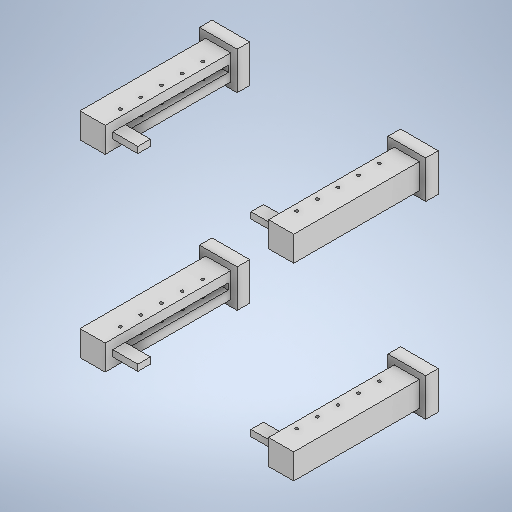
# Autodesk Inventor part: Torres
Saved by Autodesk Inventor 2026 (Build 300175050, 175E)
## iProperties
Created: 2025-04-14
Part Number: Torres
Material: Genérico
Document SubType Name: Modeling
Designer: piero
Density: 1 g/cm^3
Appearance: Valor por defecto
Author: piero
Autodesk Inventor part; units mm, degrees
ref_plane "YZ Plane" through (0, 0, 0) normal (1, 0, 0) x (0, 1, 0)
ref_plane "XZ Plane" through (0, 0, 0) normal (0, 1, 0) x (-1, 0, 0)
ref_plane "XY Plane" through (0, 0, 0) normal (0, 0, 1) x (1, 0, 0)
sketch "Boceto1" plane through (0, 0, 0) normal (0, 0, 1) x (1, 0, 0)
  line L0 (-82.5537, 351.7864) -> (67.4463, 351.7864)
  line L1 (67.4463, 351.7864) -> (67.4463, 201.7864)
  line L2 (67.4463, 201.7864) -> (-82.5537, 201.7864)
  line L3 (-82.5537, 201.7864) -> (-82.5537, 351.7864)
  line L4 (-82.5537, 351.7864) -> (67.4463, 201.7864) construction
  line L5 (67.4463, 351.7864) -> (-82.5537, 201.7864) construction
  line L6 (667.4463, 201.7864) -> (817.4463, 201.7864)
  line L7 (817.4463, 201.7864) -> (817.4463, 351.7864)
  line L8 (817.4463, 351.7864) -> (667.4463, 351.7864)
  line L9 (667.4463, 351.7864) -> (667.4463, 201.7864)
  line L10 (667.4463, 201.7864) -> (817.4463, 351.7864) construction
  line L11 (817.4463, 201.7864) -> (667.4463, 351.7864) construction
  line L12 (-82.5537, -548.2136) -> (67.4463, -548.2136)
  line L13 (67.4463, -548.2136) -> (67.4463, -398.2136)
  line L14 (67.4463, -398.2136) -> (-82.5537, -398.2136)
  line L15 (-82.5537, -398.2136) -> (-82.5537, -548.2136)
  line L16 (-82.5537, -548.2136) -> (67.4463, -398.2136) construction
  line L17 (67.4463, -548.2136) -> (-82.5537, -398.2136) construction
  line L18 (667.4463, -548.2136) -> (817.4463, -548.2136)
  line L19 (817.4463, -548.2136) -> (817.4463, -398.2136)
  line L20 (817.4463, -398.2136) -> (667.4463, -398.2136)
  line L21 (667.4463, -398.2136) -> (667.4463, -548.2136)
  line L22 (667.4463, -548.2136) -> (817.4463, -398.2136) construction
  line L23 (817.4463, -548.2136) -> (667.4463, -398.2136) construction
  point P0 (0, 0)
  point P1 (-7.5537, 276.7864)
  point P2 (742.4463, 276.7864)
  point P3 (-7.5537, -473.2136)
  point P4 (742.4463, -473.2136)
  point P5 (-7.5537, -398.2136)
  point P6 (742.4463, -398.2136)
  point P7 (667.4463, 276.7864)
  point P8 (667.4463, -473.2136)
  point P9 (67.4463, -473.2136)
  dimension "d0" = 150
  dimension "d1" = 150
  dimension "d2" = 150
  dimension "d3" = 150
  dimension "d4" = 150
  dimension "d5" = 150
  dimension "d6" = 150
  dimension "d7" = 150
  dimension "d8" = 600
  dimension "d9" = 600
  dimension "d10" = 600
  dimension "d11" = 600
  constraints: 48 end point, 13 midpoint, 8 parallel, 4 horizontal, 4 perpendicular
  measures "d0" distance of L1.end L2.end
  measures "d1" distance of L0.end L1.end
  measures "d2" distance of L8.end L7.end
  measures "d3" distance of L7.end L6.end
  measures "d4" distance of L14.end L13.end
  measures "d5" distance of L13.end L12.end
  measures "d6" distance of L20.end L19.end
  measures "d7" distance of L19.end L18.end
  measures "d8" distance from line of point (-7.554, -398.214) L2
  measures "d9" distance from line of point (742.446, -398.214) L6
  measures "d10" distance from line of point (667.446, 276.786) L1
  measures "d11" distance of point (667.446, -473.214) point (67.446, -473.214)
extrude "Extrusión1" add sketch "Boceto1" along normal blind 50
sketch "Boceto2" plane through (0, 0, 50) normal (0, 0, 1) x (1, 0, 0)
  line L0 (-57.5537, 326.7864) -> (42.4463, 326.7864)
  line L1 (42.4463, 326.7864) -> (42.4463, 226.7864)
  line L2 (42.4463, 226.7864) -> (-57.5537, 226.7864)
  line L3 (-57.5537, 226.7864) -> (-57.5537, 326.7864)
  line L4 (-57.5537, 326.7864) -> (42.4463, 226.7864) construction
  line L5 (42.4463, 326.7864) -> (-57.5537, 226.7864) construction
  line L6 (692.4463, 326.7864) -> (792.4463, 326.7864)
  line L7 (792.4463, 326.7864) -> (792.4463, 226.7864)
  line L8 (792.4463, 226.7864) -> (692.4463, 226.7864)
  line L9 (692.4463, 226.7864) -> (692.4463, 326.7864)
  line L10 (692.4463, 326.7864) -> (792.4463, 226.7864) construction
  line L11 (792.4463, 326.7864) -> (692.4463, 226.7864) construction
  line L12 (692.4463, -423.2136) -> (792.4463, -423.2136)
  line L13 (792.4463, -423.2136) -> (792.4463, -523.2136)
  line L14 (792.4463, -523.2136) -> (692.4463, -523.2136)
  line L15 (692.4463, -523.2136) -> (692.4463, -423.2136)
  line L16 (692.4463, -423.2136) -> (792.4463, -523.2136) construction
  line L17 (792.4463, -423.2136) -> (692.4463, -523.2136) construction
  line L18 (-57.5537, -523.2136) -> (42.4463, -523.2136)
  line L19 (42.4463, -523.2136) -> (42.4463, -423.2136)
  line L20 (42.4463, -423.2136) -> (-57.5537, -423.2136)
  line L21 (-57.5537, -423.2136) -> (-57.5537, -523.2136)
  line L22 (-57.5537, -523.2136) -> (42.4463, -423.2136) construction
  line L23 (42.4463, -523.2136) -> (-57.5537, -423.2136) construction
  line L24 (67.4463, 351.7864) -> (-82.5537, 351.7864) projected
  line L25 (-82.5537, 351.7864) -> (-82.5537, 201.7864) projected
  line L26 (817.4463, 351.7864) -> (667.4463, 351.7864) projected
  line L27 (667.4463, 351.7864) -> (667.4463, 201.7864) projected
  line L28 (817.4463, -398.2136) -> (667.4463, -398.2136) projected
  line L29 (-82.5537, -398.2136) -> (-82.5537, -548.2136) projected
  line L30 (67.4463, -398.2136) -> (-82.5537, -398.2136) projected
  point P0 (0, 0)
  point P1 (-7.5537, 276.7864)
  point P2 (742.4463, 276.7864)
  point P3 (742.4463, -473.2136)
  point P4 (-7.5537, -473.2136)
  point P5 (742.4463, 351.7864)
  point P6 (742.4463, 326.7864)
  point P7 (692.4463, 276.7864)
  dimension "d14" = 100
  dimension "d15" = 100
  dimension "d16" = 100
  dimension "d17" = 100
  dimension "d18" = 100
  dimension "d19" = 100
  dimension "d20" = 25
  dimension "d21" = 25
  dimension "d22" = 25
  dimension "d23" = 25
  dimension "d24" = 25
  dimension "d25" = 25
  dimension "d26" = 25
  constraints: 48 end point, 11 midpoint, 8 parallel, 4 horizontal, 4 perpendicular, 3 point on line
  measures "d14" distance of L1.end L2.end
  measures "d15" distance of L0.end L1.end
  measures "d16" distance of L7.end L8.end
  measures "d17" distance of L6.end L7.end
  measures "d18" distance of L13.end L14.end
  measures "d19" distance of L12.end L13.end
  measures "d20" distance between parallel lines of L24 L0
  measures "d21" distance between parallel lines of L25 L3
  measures "d22" distance of point (742.446, 351.786) point (742.446, 326.786)
  measures "d23" distance from line of L27 point (692.446, 276.786)
  measures "d24" distance between parallel lines of L28 L12
  measures "d25" distance between parallel lines of L29 L21
  measures "d26" distance between parallel lines of L20 L30
extrude "Extrusión2" add sketch "Boceto2" along normal blind 500
sketch "Boceto5" plane through (692.4463, 226.7864, 50) normal (-1, 0, 0) x (0, 0, 1)
  line L0 (470, 62.5) -> (420, 62.5) projected
  line L1 (470, 37.5) -> (470, 62.5) projected
  line L2 (420, 37.5) -> (470, 37.5) projected
  line L3 (420, 62.5) -> (420, 37.5) projected
  line L4 (420, 62.5) -> (470, 62.5) projected
  line L5 (470, 62.5) -> (10, 62.5)
  line L6 (10, 62.5) -> (10, 37.5)
  line L7 (10, 37.5) -> (470, 37.5)
  line L8 (470, 37.5) -> (470, 62.5)
  line L9 (470, -712.5) -> (470, -687.5) projected
  line L10 (470, -687.5) -> (10, -687.5)
  line L11 (10, -687.5) -> (10, -712.5)
  line L12 (10, -712.5) -> (470, -712.5)
  line L13 (470, -712.5) -> (470, -687.5)
  point P0 (-50, -226.7864)
  dimension "d41" = 460
  dimension "d42" = 460
  constraints: 16 end point, 4 parallel, 2 horizontal, 2 perpendicular, 1 point on line
  measures "d41" distance of L7.end L6.end
  measures "d42" distance of L12.end L11.end
extrude "Extrusión5" cut sketch "Boceto5" against normal blind 50
sketch "Boceto6" plane through (742.4463, 226.7864, 50) normal (-1, 0, 0) x (0, 0, 1)
  line L0 (470, 62.5) -> (470, 37.5) projected
  line L1 (470, 37.5) -> (10, 37.5) projected
  line L2 (470, 62.5) -> (420, 62.5)
  line L3 (420, 62.5) -> (420, 37.5)
  line L4 (420, 37.5) -> (470, 37.5)
  line L5 (470, 37.5) -> (470, 62.5)
  line L6 (10, -687.5) -> (470, -687.5) projected
  line L7 (470, -712.5) -> (10, -712.5) projected
  line L8 (470, -687.5) -> (420, -687.5)
  line L9 (420, -687.5) -> (420, -712.5)
  line L10 (420, -712.5) -> (470, -712.5)
  line L11 (470, -712.5) -> (470, -687.5)
  point P0 (-50, -226.7864)
  dimension "d45" = 50
  dimension "d46" = 50
  constraints: 16 end point, 4 parallel, 2 horizontal, 2 perpendicular, 2 point on line
  measures "d45" distance of L4.end L3.end
  measures "d46" distance of L10.end L9.end
extrude "Extrusión6" add sketch "Boceto6" along normal blind 150
sketch "Boceto7" plane through (42.4463, -523.2136, 50) normal (1, 0, 0) x (0, 0, -1)
  line L0 (-470, 37.5) -> (-420, 37.5) projected
  line L1 (-10, 62.5) -> (-420, 62.5) projected
  line L2 (-470, 37.5) -> (-10, 37.5)
  line L3 (-10, 37.5) -> (-10, 62.5)
  line L4 (-10, 62.5) -> (-470, 62.5)
  line L5 (-470, 62.5) -> (-470, 37.5)
  line L6 (-470, 787.5) -> (-420, 787.5) projected
  line L7 (-470, 787.5) -> (-10, 787.5)
  line L8 (-10, 787.5) -> (-10, 812.5)
  line L9 (-10, 812.5) -> (-470, 812.5)
  line L10 (-470, 812.5) -> (-470, 787.5)
  point P0 (50, 523.2136)
  dimension "d49" = 460
  dimension "d50" = 460
  constraints: 16 end point, 4 parallel, 2 horizontal, 2 perpendicular
  measures "d49" distance of L4.end L1.start
  measures "d50" distance of L9.end L8.end
extrude "Extrusión7" cut sketch "Boceto7" against normal blind 50
sketch "Boceto8" plane through (-7.5537, -523.2136, 50) normal (1, 0, 0) x (0, 0, -1)
  line L0 (-470, 62.5) -> (-470, 37.5) projected
  line L1 (-420, 62.5) -> (-470, 62.5) projected
  line L2 (-470, 37.5) -> (-420, 37.5)
  line L3 (-420, 37.5) -> (-420, 62.5)
  line L4 (-420, 62.5) -> (-470, 62.5)
  line L5 (-470, 62.5) -> (-470, 37.5)
  line L6 (-470, 787.5) -> (-420, 787.5) projected
  line L7 (-470, 812.5) -> (-420, 812.5) projected
  line L8 (-470, 787.5) -> (-420, 787.5)
  line L9 (-420, 787.5) -> (-420, 812.5)
  line L10 (-420, 812.5) -> (-470, 812.5)
  line L11 (-470, 812.5) -> (-470, 787.5)
  point P0 (50, 523.2136)
  dimension "d53" = 50
  dimension "d54" = 50
  constraints: 16 end point, 4 parallel, 2 horizontal, 2 perpendicular
  measures "d53" distance of L4.end L1.start
  measures "d54" distance of L10.end L7.end
extrude "Extrusión8" add sketch "Boceto8" along normal blind 150
sketch "Boceto9" plane through (-57.5537, -523.2136, 50) normal (0, -1, 0) x (1, 0, 0)
  line L0 (50, 420) -> (100, 420) projected
  circle A0 centre (74, 414) radius 6
  circle A1 centre (74, 332) radius 6
  circle A2 centre (74, 250) radius 6
  circle A3 centre (74, 168) radius 6
  circle A4 centre (74, 86) radius 6
  line L1 (100, 0) -> (100, 500) projected
  circle A5 centre (776, 414) radius 6
  line L2 (750, 420) -> (800, 420) projected
  line L3 (750, 0) -> (750, 500) projected
  circle A6 centre (776, 332) radius 6
  circle A7 centre (776, 250) radius 6
  circle A8 centre (776, 168) radius 6
  circle A9 centre (776, 86) radius 6
  line L4 (725, 0) -> (875, 0) projected
  point P0 (57.5537, -50)
  dimension "d60" = 12
  dimension "d61" = 0
  dimension "d62" = 12
  dimension "d63" = 70
  dimension "d64" = 12
  dimension "d65" = 12
  dimension "d66" = 12
  dimension "d69" = 82
  dimension "d70" = 70
  dimension "d71" = 82
  dimension "d74" = 20
  dimension "d75" = 12
  dimension "d76" = 0
  dimension "d77" = 20
  dimension "d78" = 12
  dimension "d83" = 82
  dimension "d84" = 12
  dimension "d85" = 82
  dimension "d86" = 12
  dimension "d87" = 70
  dimension "d88" = 12
  dimension "d89" = 82
  constraints: 10 centre point
  measures "d60" diameter of A0
  measures "d61" distance edge to line of A0 L0
  measures "d62" diameter of A1
  measures "d64" diameter of A2
  measures "d65" diameter of A3
  measures "d66" diameter of A4
  measures "d69" distance of A2.centre A1.centre
  measures "d71" distance of A4.centre A3.centre
  measures "d74" distance edge to line of A0 L1
  measures "d75" diameter of A5
  measures "d76" distance edge to line of A5 L2
  measures "d77" distance edge to line of A5 L3
  measures "d78" diameter of A6
  measures "d83" distance of A6.centre A5.centre
  measures "d84" diameter of A7
  measures "d85" distance of A7.centre A6.centre
  measures "d86" diameter of A8
  measures "d88" diameter of A9
  measures "d89" distance of A9.centre A8.centre
hole "Agujero1" at (16.4463, -523.2136, 464) direction (0, 1, 0) diameter 11.835 depth 100 thread size "M14x2" class "6H" standard "ISO Metric profile"
hole "Agujero2" at (16.4463, -523.2136, 382) direction (0, 1, 0) diameter 11.835 depth 100 thread size "M14x2" class "6H" standard "ISO Metric profile"
hole "Agujero3" at (16.4463, -523.2136, 300) direction (0, 1, 0) diameter 11.835 depth 100 thread size "M14x2" class "6H" standard "ISO Metric profile"
hole "Agujero4" at (16.4463, -523.2136, 218) direction (0, 1, 0) diameter 11.835 depth 100 thread size "M14x2" class "6H" standard "ISO Metric profile"
hole "Agujero5" at (16.4463, -523.2136, 136) direction (0, 1, 0) diameter 11.835 depth 100 thread size "M14x2" class "6H" standard "ISO Metric profile"
hole "Agujero6" at (718.4463, -523.2136, 464) direction (0, 1, 0) diameter 11.835 depth 100 thread size "M14x2" class "6H" standard "ISO Metric profile"
hole "Agujero7" at (718.4463, -523.2136, 382) direction (0, 1, 0) diameter 11.835 depth 100 thread size "M14x2" class "6H" standard "ISO Metric profile"
hole "Agujero8" at (718.4463, -523.2136, 300) direction (0, 1, 0) diameter 11.835 depth 100 thread size "M14x2" class "6H" standard "ISO Metric profile"
hole "Agujero9" at (718.4463, -523.2136, 218) direction (0, 1, 0) diameter 11.835 depth 100 thread size "M14x2" class "6H" standard "ISO Metric profile"
hole "Agujero10" at (718.4463, -523.2136, 136) direction (0, 1, 0) diameter 11.835 depth 100 thread size "M14x2" class "6H" standard "ISO Metric profile"
sketch "Boceto10" plane through (692.4463, 326.7864, 50) normal (0, 1, 0) x (1, 0, 0)
  line L0 (50, -420) -> (0, -420) projected
  circle A0 centre (26, -414) radius 5.9175 projected
  circle A1 centre (26, -414) radius 6
  circle A2 centre (26, -332) radius 5.9175 projected
  circle A3 centre (26, -332) radius 6
  circle A4 centre (26, -250) radius 5.9175 projected
  circle A5 centre (26, -250) radius 6
  circle A6 centre (26, -168) radius 5.9175 projected
  circle A7 centre (26, -168) radius 6
  circle A8 centre (26, -86) radius 5.9175 projected
  circle A9 centre (26, -86) radius 6
  circle A10 centre (-676, -414) radius 5.9175 projected
  circle A11 centre (-676, -414) radius 6
  circle A12 centre (-676, -332) radius 5.9175 projected
  circle A13 centre (-676, -332) radius 6
  circle A14 centre (-676, -250) radius 5.9175 projected
  circle A15 centre (-676, -250) radius 6
  circle A16 centre (-676, -168) radius 5.9175 projected
  circle A17 centre (-676, -168) radius 6
  circle A18 centre (-676, -86) radius 5.9175 projected
  circle A19 centre (-676, -86) radius 6
  point P0 (-692.4463, 50)
  dimension "d161" = 12
  dimension "d162" = 12
  dimension "d163" = 12
  dimension "d164" = 12
  dimension "d165" = 12
  dimension "d166" = 12
  dimension "d167" = 12
  dimension "d168" = 12
  dimension "d169" = 12
  dimension "d170" = 12
  constraints: 10 centre point, 10 coincident
  measures "d161" diameter of A1
  measures "d162" diameter of A3
  measures "d163" diameter of A5
  measures "d164" diameter of A7
  measures "d165" diameter of A9
  measures "d166" diameter of A11
  measures "d167" diameter of A13
  measures "d168" diameter of A15
  measures "d169" diameter of A17
  measures "d170" diameter of A19
hole "Agujero11" at (718.4463, 326.7864, 464) direction (0, -1, 0) diameter 11.835 depth 100 thread size "M14x2" class "6H" standard "ISO Metric profile"
hole "Agujero12" at (718.4463, 326.7864, 382) direction (0, -1, 0) diameter 11.835 depth 100 thread size "M14x2" class "6H" standard "ISO Metric profile"
hole "Agujero13" at (718.4463, 326.7864, 300) direction (0, -1, 0) diameter 11.835 depth 100 thread size "M14x2" class "6H" standard "ISO Metric profile"
hole "Agujero14" at (718.4463, 326.7864, 218) direction (0, -1, 0) diameter 11.835 depth 100 thread size "M14x2" class "6H" standard "ISO Metric profile"
hole "Agujero15" at (718.4463, 326.7864, 136) direction (0, -1, 0) diameter 11.835 depth 100 thread size "M14x2" class "6H" standard "ISO Metric profile"
hole "Agujero16" at (16.4463, 326.7864, 464) direction (0, -1, 0) diameter 11.835 depth 100 thread size "M14x2" class "6H" standard "ISO Metric profile"
hole "Agujero17" at (16.4463, 326.7864, 382) direction (0, -1, 0) diameter 11.835 depth 100 thread size "M14x2" class "6H" standard "ISO Metric profile"
hole "Agujero18" at (16.4463, 326.7864, 300) direction (0, -1, 0) diameter 11.835 depth 100 thread size "M14x2" class "6H" standard "ISO Metric profile"
hole "Agujero19" at (16.4463, 326.7864, 218) direction (0, -1, 0) diameter 11.835 depth 100 thread size "M14x2" class "6H" standard "ISO Metric profile"
hole "Agujero20" at (16.4463, 326.7864, 136) direction (0, -1, 0) diameter 11.835 depth 100 thread size "M14x2" class "6H" standard "ISO Metric profile"
sketch "Boceto11" plane through (-7.5537, -485.7136, 470) normal (0, 0, -1) x (-1, 0, 0)
  circle A0 centre (-120, 12.5) radius 5
  line L0 (-150, 0) -> (-150, 25) projected
  circle A1 centre (-120, 762.5) radius 5
  line L1 (-150, 750) -> (-150, 775) projected
  line L2 (-50, 0) -> (-150, 0) projected
  line L3 (-50, 750) -> (-150, 750) projected
  circle A2 centre (-630, 762.5) radius 5
  line L4 (-600, 775) -> (-600, 750) projected
  line L5 (-700, 750) -> (-600, 750) projected
  circle A3 centre (-630, 12.5) radius 5
  line L6 (-600, 25) -> (-600, 0) projected
  line L7 (-700, 0) -> (-600, 0) projected
  point P0 (-7.5537, 485.7136)
  point P1 (-150, 12.5)
  point P2 (-150, 762.5)
  point P3 (-600, 762.5)
  point P4 (-600, 12.5)
  dimension "d241" = 10
  dimension "d242" = 30
  dimension "d243" = 10
  dimension "d244" = 30
  dimension "d245" = 12.5
  dimension "d246" = 12.5
  dimension "d247" = 10
  dimension "d248" = 30
  dimension "d249" = 12.5
  dimension "d250" = 10
  dimension "d251" = 30
  dimension "d252" = 12.5
  constraints: 4 centre point, 4 midpoint
  measures "d241" diameter of A0
  measures "d242" distance of point (-150, 12.5) A0.centre
  measures "d243" diameter of A1
  measures "d244" distance of A1.centre point (-150, 762.5)
  measures "d245" distance from line of L2 A0.centre
  measures "d246" distance from line of L3 A1.centre
  measures "d247" diameter of A2
  measures "d248" distance of A2.centre point (-600, 762.5)
  measures "d249" distance from line of L5 A2.centre
  measures "d250" diameter of A3
  measures "d251" distance of point (-600, 12.5) A3.centre
  measures "d252" distance from line of L7 A3.centre
hole "Agujero21" at (622.4463, -473.2136, 470) direction (0, 0, 1) diameter 10.106 depth 25 thread size "M12x1.75" class "6H" standard "ISO Metric profile"
hole "Agujero22" at (622.4463, 276.7864, 470) direction (0, 0, 1) diameter 10.106 depth 25 thread size "M12x1.75" class "6H" standard "ISO Metric profile"
hole "Agujero23" at (112.4463, 276.7864, 470) direction (0, 0, 1) diameter 10.106 depth 25 thread size "M12x1.75" class "6H" standard "ISO Metric profile"
hole "Agujero24" at (112.4463, -473.2136, 470) direction (0, 0, 1) diameter 10.106 depth 25 thread size "M12x1.75" class "6H" standard "ISO Metric profile"
